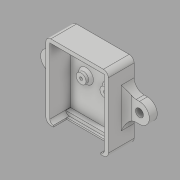
# Autodesk Inventor part: TOF Case P1
Saved by Autodesk Inventor 2019.3 (Build 233278000, 278)
## iProperties
Created: 2019-02-11
Part Number: TOF Case P1
Material: Generic
Document SubType Name: Modeling
Designer: erics
Density: 1 g/cm^3
Appearance: Default
Mass: 13.2352 g
Surface Area: 94.1174 cm^2
Volume: 13.2352 cm^3
Author: erics
Autodesk Inventor part; units mm, degrees
ref_plane "YZ Plane" through (0, 0, 0) normal (1, 0, 0) x (0, 1, 0)
ref_plane "XZ Plane" through (0, 0, 0) normal (0, 1, 0) x (-1, 0, 0)
ref_plane "XY Plane" through (0, 0, 0) normal (0, 0, 1) x (1, 0, 0)
sketch "Sketch1" plane through (0, 0, 0) normal (0, 0, 1) x (1, 0, 0)
  line L0 (0, 0) -> (40.132, 0)
  line L1 (40.132, 0) -> (40.132, 48.26)
  line L2 (40.132, 48.26) -> (0, 48.26)
  line L3 (0, 48.26) -> (0, 0)
  line L4 (3.556, 44.704) -> (36.576, 44.704) construction
  line L5 (36.576, 44.704) -> (36.576, 1.524) construction
  line L6 (36.576, 1.524) -> (3.556, 1.524) construction
  line L7 (3.556, 1.524) -> (3.556, 44.704) construction
  line L8 (37.592, 1.016) -> (37.592, 45.72)
  line L9 (37.592, 45.72) -> (2.54, 45.72)
  line L10 (2.54, 45.72) -> (2.54, 1.016)
  line L11 (2.54, 1.016) -> (37.592, 1.016) construction
  line L12 (2.54, 1.016) -> (2.54, 0)
  line L13 (37.592, 1.016) -> (37.592, 0)
  line L14 (12.446, 25.654) -> (27.686, 25.654)
  point P0 (20.066, 48.26)
  point P1 (20.066, 44.704)
  point P2 (3.556, 23.114)
  point P3 (0, 24.13)
  point P4 (20.066, 25.654)
  dimension "d2" = 33.02
  dimension "d3" = 43.18
  dimension "d4" = 1.524
  dimension "d8" = 2.54
  dimension "d9" = 1.016
  dimension "d14" = 15.24
  dimension "d15" = 19.05
  dimension "d34" = 1.016
  dimension "d35" = 1.016
  constraints: 30 end point, 5 midpoint, 5 parallel, 4 horizontal, 4 perpendicular, 2 point on line, 2 vertical alignment, 2 other
  measures "d2" distance of L5.end L6.end
  measures "d3" distance of L4.end L5.end
  measures "d4" distance between parallel lines of L6 L0
  measures "d8" distance between parallel lines of L3 L10
  measures "d9" distance between parallel lines of L11 L0
  measures "d14" distance of L14.start L14.end
  measures "d15" distance between parallel lines of L4 L14
  measures "d34" distance between parallel lines of L9 L4
  measures "d35" distance between parallel lines of L7 L10
extrude "Extrusion1" add sketch "Sketch1" against normal blind 3.175
sketch "Sketch2" plane through (0, 0, 0) normal (0, 0, 1) x (1, 0, 0)
  line L0 (2.54, 1.016) -> (2.54, 0) projected
  line L1 (0, 48.26) -> (0, 0) projected
  line L2 (2.54, 45.72) -> (2.54, 1.016) projected
  line L3 (37.592, 45.72) -> (2.54, 45.72) projected
  line L4 (40.132, 48.26) -> (0, 48.26) projected
  line L5 (40.132, 0) -> (40.132, 48.26) projected
  line L6 (37.592, 1.016) -> (37.592, 0) projected
  line L7 (37.592, 1.016) -> (37.592, 45.72) projected
  line L8 (0, 0) -> (2.54, 0)
  line L9 (37.592, 0) -> (40.132, 0)
  constraints: 4 end point, 1 horizontal
extrude "Extrusion2" add sketch "Sketch2" along normal blind 13.3856
sketch "Sketch3" plane through (0, 0, 0) normal (0, 0, 1) x (1, 0, 0)
  line L0 (2.54, 1.016) -> (37.592, 1.016) projected
  line L1 (2.54, 0) -> (37.592, 0) projected
  line L2 (2.54, 0) -> (2.54, 45.72) projected
  line L3 (37.592, 45.72) -> (37.592, 0) projected
  point P0 (0, 0)
extrude "Extrusion3" add sketch "Sketch3" along normal blind 4.775
sketch "Sketch4" plane through (0, 0, 0) normal (0, 0, 1) x (1, 0, 0)
  circle A0 centre (12.446, 25.654) radius 3.175
  circle A1 centre (27.686, 25.654) radius 3.175
  circle A2 centre (12.446, 25.654) radius 0.9652
  circle A3 centre (27.686, 25.654) radius 0.9652
  point P0 (0, 0)
  dimension "d16" = 6.35
  dimension "d18" = 1.9304
  constraints: 4 centre point, 4 coincident, 2 equal radius
  measures "d16" diameter of A0
  measures "d18" diameter of A2
extrude "Extrusion4" add sketch "Sketch4" along normal blind 3.175
extrude "Extrusion8" cut sketch "Sketch4" against normal through all contours A2 | A3
sketch "Sketch5" plane through (0, 0, 0) normal (0, 0, 1) x (1, 0, 0)
  circle A0 centre (12.446, 25.654) radius 3.175 construction
  circle A1 centre (27.686, 25.654) radius 3.175 construction
  line L0 (2.54, 1.016) -> (37.592, 1.016) construction
  line L1 (37.592, 1.016) -> (37.592, 45.72) construction
  line L2 (37.592, 45.72) -> (2.54, 45.72) construction
  line L3 (2.54, 45.72) -> (2.54, 1.016) construction
  line L4 (3.556, 44.704) -> (36.576, 44.704) construction
  line L5 (3.556, 1.524) -> (3.556, 44.704) construction
  line L6 (36.576, 44.704) -> (36.576, 1.524) construction
  line L7 (36.576, 1.524) -> (3.556, 1.524) construction
  line L8 (2.54, 1.016) -> (37.592, 1.016)
  line L9 (37.592, 1.016) -> (37.592, 3.048)
  line L10 (37.592, 3.048) -> (2.54, 3.048)
  line L11 (2.54, 3.048) -> (2.54, 1.016)
  line L12 (2.54, 45.72) -> (37.592, 45.72)
  line L13 (37.592, 45.72) -> (37.592, 43.18)
  line L14 (37.592, 43.18) -> (2.54, 43.18)
  line L15 (2.54, 43.18) -> (2.54, 45.72)
  point P0 (0, 0)
  dimension "d21" = 1.524
  dimension "d25" = 1.524
  constraints: 16 end point, 4 parallel, 2 horizontal, 2 perpendicular, 2 point on line
  measures "d21" distance between parallel lines of L10 L7
  measures "d25" distance between parallel lines of L4 L14
extrude "Extrusion5" add sketch "Sketch5" along normal blind 3.175
sketch "Sketch6" plane through (0, 0, 4.775) normal (0, 0, 1) x (1, 0, 0)
  line L0 (40.132, 0) -> (0, 0) construction
  line L1 (4.826, 0) -> (2.54, 0)
  line L2 (2.54, 0) -> (2.54, 1.016)
  line L3 (2.54, 1.016) -> (4.826, 1.016)
  line L4 (4.826, 1.016) -> (4.826, 0)
  line L5 (2.54, 0) -> (2.54, 45.72) projected
  line L6 (37.592, 1.016) -> (2.54, 1.016) construction
  line L7 (35.306, 0) -> (37.592, 0)
  line L8 (37.592, 0) -> (37.592, 1.016)
  line L9 (37.592, 1.016) -> (35.306, 1.016)
  line L10 (35.306, 1.016) -> (35.306, 0)
  dimension "d26" = 2.286
  dimension "d27" = 2.286
  constraints: 16 end point, 4 parallel, 4 point on line, 2 horizontal, 2 perpendicular
  measures "d26" distance between parallel lines of L4 L2
  measures "d27" distance between parallel lines of L8 L10
extrude "Extrusion6" add sketch "Sketch6" along normal up to surface (8.6106 mm away)
fillet "Fillet1" radius 2.286 2 edges at (37.592, 1.016, 8.2803) (2.54, 1.016, 8.2803)
chamfer "Chamfer2" distance 1.524 angle 45 2 edges at (9.271, 25.654, 0) (24.511, 25.654, 0)
fillet "Fillet2" radius 3.175 4 edges at (0, 0, 5.1053) (40.132, 0, 5.1053) (40.132, 48.26, 5.1053) (0, 48.26, 5.1053)
sketch "Sketch7" plane through (0, 0, -3.175) normal (0, 0, -1) x (-1, 0, 0)
  circle A0 centre (8.509, 24.13) radius 2.5527
  line L0 (-3.175, 48.26) -> (-36.957, 48.26) construction
  line L1 (-40.132, 45.085) -> (-40.132, 3.175) construction
  line L2 (-36.957, 0) -> (-3.175, 0) construction
  line L3 (0, 3.175) -> (0, 45.085) construction
  line L4 (-40.132, 48.26) -> (0, 48.26) construction
  line L5 (-20.066, 48.26) -> (-20.066, 0) construction
  arc A1 (0, 36.83) -> (6.35, 30.48) centre (6.35, 36.83) ccw
  arc A2 (6.35, 17.78) -> (0, 11.43) centre (6.35, 11.43) ccw
  line L6 (6.35, 30.48) -> (8.509, 30.48)
  arc A3 (8.509, 17.78) -> (8.509, 30.48) centre (8.509, 24.13) ccw
  line L7 (8.509, 17.78) -> (6.35, 17.78)
  line L8 (0, 36.83) -> (0, 11.43)
  line L9 (0, 0) -> (0, 48.26) projected
  circle A4 centre (-48.641, 24.13) radius 2.5527
  arc A5 (-46.482, 30.48) -> (-40.132, 36.83) centre (-46.482, 36.83) ccw
  arc A6 (-40.132, 11.43) -> (-46.482, 17.78) centre (-46.482, 11.43) ccw
  line L10 (-46.482, 30.48) -> (-48.641, 30.48)
  arc A7 (-48.641, 30.48) -> (-48.641, 17.78) centre (-48.641, 24.13) ccw
  line L11 (-48.641, 17.78) -> (-46.482, 17.78)
  line L12 (-40.132, 36.83) -> (-40.132, 11.43)
  arc A8 (0, 45.085) -> (-3.175, 48.26) centre (-3.175, 45.085) ccw projected
  arc A9 (-36.957, 48.26) -> (-40.132, 45.085) centre (-36.957, 45.085) ccw projected
  arc A10 (-40.132, 3.175) -> (-36.957, 0) centre (-36.957, 3.175) ccw projected
  arc A11 (-3.175, 0) -> (0, 3.175) centre (-3.175, 3.175) ccw projected
  point P0 (-3.175, 48.26)
  point P1 (0, 24.13)
  point P2 (-40.132, 24.13)
  dimension "d40" = 5.1054
  dimension "d41" = 6.35
  dimension "d43" = 6.35
  dimension "d44" = 57.15
  constraints: 14 end point, 12 point on circle, 11 symmetric about line, 8 centre point, 7 tangent, 3 midpoint, 2 coincident, 2 horizontal, 2 point on line, 1 collinear, 1 equal radius, 1 horizontal alignment, 4 other
  measures "d40" diameter of A0
  measures "d41" radius of A3
  measures "d43" radius of A1
  measures "d44" distance of A0.centre A4.centre
extrude "Extrusion7" add sketch "Sketch7" against normal blind 5.08
fillet "Fillet3" radius 3.175 2 edges at (40.132, 24.13, 1.905) (0, 24.13, 1.905)
equation "\"d12\" = BoardOffset + PCBThickness"
equation "\"d19\" = BoardOffset"
equation "\"d23\" = BoardOffset"
equation "\"d27\" = d26"
equation "\"d28\" = BoardOffset"
equation "\"PCBThickness\" = 1.6"
equation "\"BoardOffset\" = 3.175"
body "Solid1"
